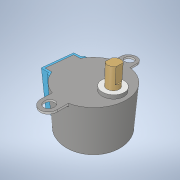
# Autodesk Inventor part: Stepper 28BYJ-48
Saved by Autodesk Inventor 2021.1 (Build 251245010, 245A)
## iProperties
Created: 2020-12-02
Part Number: Stepper 28BYJ-48
Material: Типовые
Document SubType Name: Modeling
Designer: Администратор
Density: 1 g/cm^3
Appearance: По умолчанию
Author: Администратор
Autodesk Inventor part; units mm, degrees
ref_plane "YZ Plane" through (0, 0, 0) normal (1, 0, 0) x (0, 1, 0)
ref_plane "XZ Plane" through (0, 0, 0) normal (0, 1, 0) x (-1, 0, 0)
ref_plane "XY Plane" through (0, 0, 0) normal (0, 0, 1) x (1, 0, 0)
sketch "Эскиз1" plane through (0, 0, 0) normal (0, 1, 0) x (-1, 0, 0)
  circle A0 centre (0, 0) radius 14
  dimension "d0" = 28
  constraints: 1 centre point, 1 coincident
  measures "d0" diameter of A0
extrude "Выдавливание1" add sketch "Эскиз1" along normal blind 19
sketch "Эскиз2" plane through (0, 19, 0) normal (0, 1, 0) x (1, 0, 0)
  circle A0 centre (8, 0) radius 4.5
  point P0 (0, 0)
  dimension "d3" = 9
  dimension "d4" = 8
  constraints: 1 centre point
  measures "d3" diameter of A0
  measures "d4" distance of point (0, 0) A0.centre
extrude "Выдавливание2" add sketch "Эскиз2" along normal blind 1.5
sketch "Эскиз3" plane through (8, 20.5, 0) normal (0, 1, 0) x (1, 0, 0)
  circle A0 centre (0, 0) radius 2.5
  point P0 (-8, 0)
  dimension "d7" = 5
  constraints: 1 centre point
  measures "d7" diameter of A0
extrude "Выдавливание3" add sketch "Эскиз3" along normal blind 8
sketch "Эскиз4" plane through (8, 28.5, 0) normal (0, 1, 0) x (1, 0, 0)
  circle A0 centre (0, 0) radius 2.5 projected
  line L0 (2, 1.5) -> (2, -1.5)
  line L1 (-2, -1.5) -> (-2, 1.5)
  point P0 (-8, 0)
  dimension "d12" = 3
  dimension "d13" = 3
  constraints: 4 end point, 4 point on circle, 1 parallel, 1 vertical
  measures "d12" distance of L0.start L0.end
  measures "d13" distance of L1.start L1.end
extrude "Выдавливание4" cut sketch "Эскиз4" against normal blind 6 contours A0 L0 | L1 A0
sketch "Эскиз5" plane through (0, 19, 0) normal (0, 1, 0) x (1, 0, 0)
  arc A0 (-3.5, -17.5) -> (3.5, -17.5) centre (0, -17.5) ccw
  arc A1 (3.5, 17.5) -> (-3.5, 17.5) centre (0, 17.5) ccw
  circle A2 centre (0, 0) radius 14 projected
  line L0 (-3.5, -17.5) -> (-3.5, -13.5554)
  line L1 (3.5, 17.5) -> (3.5, 13.5554)
  line L2 (-3.5, 17.5) -> (-3.5, 13.5554)
  line L3 (3.5, -17.5) -> (3.5, -13.5554)
  line L4 (0, 29.4009) -> (0, -29.4054) construction
  circle A3 centre (8, 0) radius 4.5 projected
  dimension "d16" = 7
  dimension "d17" = 17.5
  dimension "d18" = 7
  dimension "d19" = 17.5
  dimension "d41" = 8
  constraints: 10 point on circle, 8 end point, 4 point on line, 4 tangent, 3 vertical, 2 centre point, 1 parallel
  measures "d16" diameter of A0
  measures "d17" distance of point (0, 0) A0.centre
  measures "d18" diameter of A1
  measures "d19" distance of point (0, 0) A1.centre
  measures "d41" distance from line of A3.centre L4
extrude "Выдавливание5" add sketch "Эскиз5" against normal blind 0.8 contours L0 A2 L3 A0 | L2 A1 L1 A2
sketch "Эскиз6" plane through (0, 19, 0) normal (0, 1, 0) x (1, 0, 0)
  circle A0 centre (0, 17.5) radius 2.1
  circle A1 centre (0, -17.5) radius 2.1
  point P0 (0, 0)
  dimension "d22" = 4.2
  dimension "d23" = 4.2
  dimension "d24" = 17.5
  dimension "d25" = 17.5
  constraints: 2 centre point
  measures "d22" diameter of A0
  measures "d23" diameter of A1
  measures "d24" distance of point (0, 0) A0.centre
  measures "d25" distance of point (0, 0) A1.centre
extrude "Выдавливание6" cut sketch "Эскиз6" against normal blind 0.8
fillet "Сопряжение1" radius 0.5 1 edges at (14, 0, 0)
fillet "Сопряжение2" radius 0.5 1 edges at (0, 18.2, -14)
fillet "Сопряжение3" radius 0.5 1 edges at (0, 18.2, 14)
sketch "Эскиз7" plane through (0, 19, 0) normal (0, 1, 0) x (1, 0, 0)
  line L0 (-17, -7.3) -> (-17, 7.3)
  line L1 (0, 0) -> (-17, 0) construction
  line L2 (-13.1038, 7.3) -> (-17, 7.3)
  line L3 (-13.1038, -7.3) -> (-17, -7.3)
  arc A0 (-3.5, 13.5554) -> (-3.5, -13.5554) centre (0, 0) ccw projected
  line L4 (-12.5024, -6.3) -> (-16, -6.3)
  line L5 (-16, -6.3) -> (-16, 6.3)
  line L6 (-16, 6.3) -> (-12.5024, 6.3)
  line L7 (-11.2743, 8.3) -> (-12.4944, 8.3)
  line L8 (-12.4944, -8.3) -> (-11.2743, -8.3)
  arc A1 (-12.4944, 8.3) -> (-13.1038, 7.3) centre (0, 0) ccw
  arc A2 (-13.1038, -7.3) -> (-12.4944, -8.3) centre (0, 0) ccw
  point P0 (0, 7.4186)
  point P1 (0, -7.4186)
  point P2 (-11.9461, 7.3)
  point P3 (-11.9461, -7.3)
  dimension "d31" = 17
  dimension "d32" = 14.6
  dimension "d33" = 1
  dimension "d35" = 1
  constraints: 18 end point, 10 point on circle, 3 perpendicular, 2 centre point, 2 coincident, 2 symmetric about line, 1 midpoint, 1 vertical
  measures "d31" distance from line of L0 L1.start
  measures "d32" distance between parallel lines of L3 L2
  measures "d33" distance between parallel lines of L3 L4
  measures "d35" distance between parallel lines of L2 L7
extrude "Выдавливание7" add sketch "Эскиз7" against normal blind 17 separate body contours L0 L2 A1 L7 A0 L6 L5 L4 L8 A2 L3
sketch "Эскиз9" plane through (0, 19, 0) normal (0, 1, 0) x (1, 0, 0)
  arc A0 (-3.5, 13.5554) -> (-3.5, -13.5554) centre (0, 0) ccw projected
  line L0 (-3.5, 13.5554) -> (-3.5, 17.5) projected
  arc A1 (3.5, 17.5) -> (-3.5, 17.5) centre (0, 17.5) ccw projected
  line L1 (3.5, 17.5) -> (3.5, 13.5554) projected
  arc A2 (3.5, -13.5554) -> (3.5, 13.5554) centre (0, 0) ccw projected
  line L2 (3.5, -13.5554) -> (3.5, -17.5) projected
  arc A3 (-3.5, -17.5) -> (3.5, -17.5) centre (0, -17.5) ccw projected
  line L3 (-3.5, -17.5) -> (-3.5, -13.5554) projected
  circle A4 centre (0, 17.5) radius 2.1 projected
  circle A5 centre (0, -17.5) radius 2.1 projected
  circle A6 centre (8, 0) radius 4.5 projected
  arc A7 (-13.1038, -7.3) -> (-12.4944, -8.3) centre (0, 0) ccw projected
  line L4 (-13.1038, -7.3) -> (-17, -7.3) projected
  line L5 (-17, -7.3) -> (-17, 7.3) projected
  line L6 (-17, 7.3) -> (-13.1038, 7.3) projected
  arc A8 (-12.4944, 8.3) -> (-13.1038, 7.3) centre (0, 0) ccw projected
  line L7 (-12.4944, 8.3) -> (-11.2743, 8.3) projected
  arc A9 (-11.2743, 8.3) -> (-12.5024, 6.3) centre (0, 0) ccw projected
  line L8 (-12.5024, 6.3) -> (-16, 6.3) projected
  line L9 (-16, 6.3) -> (-16, -6.3) projected
  line L10 (-16, -6.3) -> (-12.5024, -6.3) projected
  arc A10 (-12.5024, -6.3) -> (-11.2743, -8.3) centre (0, 0) ccw projected
  line L11 (-11.2743, -8.3) -> (-12.4944, -8.3) projected
  arc A11 (-3.5, 13.5554) -> (-3.5, -13.5554) centre (0, 0) ccw projected
  line L12 (-3.5, 13.5554) -> (-3.5, 17.5) projected
  line L13 (-3.5, -17.5) -> (-3.5, -13.5554) projected
  circle A12 centre (0, 17.5) radius 2.1 projected
  circle A13 centre (0, -17.5) radius 2.1 projected
  circle A14 centre (8, 0) radius 4.5 projected
  arc A15 (-13.1038, -7.3) -> (-12.4944, -8.3) centre (0, 0) ccw projected
  line L14 (-13.1038, -7.3) -> (-17, -7.3) projected
  line L15 (-17, -7.3) -> (-17, 7.3) projected
  line L16 (-17, 7.3) -> (-13.1038, 7.3) projected
  arc A16 (-12.4944, 8.3) -> (-13.1038, 7.3) centre (0, 0) ccw projected
  line L17 (-12.4944, 8.3) -> (-11.2743, 8.3) projected
  arc A17 (-11.2743, 8.3) -> (-12.5024, 6.3) centre (0, 0) ccw projected
  line L18 (-12.5024, 6.3) -> (-16, 6.3) projected
  line L19 (-16, 6.3) -> (-16, -6.3) projected
  line L20 (-16, -6.3) -> (-12.5024, -6.3) projected
  arc A18 (-12.5024, -6.3) -> (-11.2743, -8.3) centre (0, 0) ccw projected
  line L21 (-11.2743, -8.3) -> (-12.4944, -8.3) projected
  arc A19 (-3.5, 13.5554) -> (-3.5, -13.5554) centre (0, 0) ccw projected
  line L22 (-3.5, 13.5554) -> (-3.5, 17.5) projected
  line L23 (-3.5, -17.5) -> (-3.5, -13.5554) projected
  circle A20 centre (0, 17.5) radius 2.1 projected
  circle A21 centre (0, -17.5) radius 2.1 projected
  circle A22 centre (8, 0) radius 4.5 projected
  arc A23 (-13.1038, -7.3) -> (-12.4944, -8.3) centre (0, 0) ccw projected
  line L24 (-13.1038, -7.3) -> (-17, -7.3) projected
  line L25 (-17, -7.3) -> (-17, 7.3) projected
  line L26 (-17, 7.3) -> (-13.1038, 7.3) projected
  arc A24 (-12.4944, 8.3) -> (-13.1038, 7.3) centre (0, 0) ccw projected
  line L27 (-12.4944, 8.3) -> (-11.2743, 8.3) projected
  arc A25 (-11.2743, 8.3) -> (-12.5024, 6.3) centre (0, 0) ccw projected
  line L28 (-12.5024, 6.3) -> (-16, 6.3) projected
  line L29 (-16, 6.3) -> (-16, -6.3) projected
  line L30 (-16, -6.3) -> (-12.5024, -6.3) projected
  arc A26 (-12.5024, -6.3) -> (-11.2743, -8.3) centre (0, 0) ccw projected
  line L31 (-11.2743, -8.3) -> (-12.4944, -8.3) projected
  arc A27 (-3.5, 13.5554) -> (-3.5, -13.5554) centre (0, 0) ccw projected
  line L32 (-3.5, 13.5554) -> (-3.5, 17.5) projected
  line L33 (-3.5, -17.5) -> (-3.5, -13.5554) projected
  circle A28 centre (0, 17.5) radius 2.1 projected
  circle A29 centre (0, -17.5) radius 2.1 projected
  circle A30 centre (8, 0) radius 4.5 projected
  arc A31 (-13.1038, -7.3) -> (-12.4944, -8.3) centre (0, 0) ccw projected
  line L34 (-13.1038, -7.3) -> (-17, -7.3) projected
  line L35 (-17, -7.3) -> (-17, 7.3) projected
  line L36 (-17, 7.3) -> (-13.1038, 7.3) projected
  arc A32 (-12.4944, 8.3) -> (-13.1038, 7.3) centre (0, 0) ccw projected
  line L37 (-12.4944, 8.3) -> (-11.2743, 8.3) projected
  arc A33 (-11.2743, 8.3) -> (-12.5024, 6.3) centre (0, 0) ccw projected
  line L38 (-12.5024, 6.3) -> (-16, 6.3) projected
  line L39 (-16, 6.3) -> (-16, -6.3) projected
  line L40 (-16, -6.3) -> (-12.5024, -6.3) projected
  arc A34 (-12.5024, -6.3) -> (-11.2743, -8.3) centre (0, 0) ccw projected
  line L41 (-11.2743, -8.3) -> (-12.4944, -8.3) projected
  arc A35 (-3.5, 13.5554) -> (-3.5, -13.5554) centre (0, 0) ccw projected
  line L42 (-16, 6.3) -> (-12.5024, 6.3) projected
  line L43 (-16, -6.3) -> (-16, 6.3) projected
  circle A36 centre (0, 17.5) radius 2.1 projected
  circle A37 centre (0, -17.5) radius 2.1 projected
  circle A38 centre (8, 0) radius 4.5 projected
  arc A39 (-3.5, 13.5554) -> (-3.5, -13.5554) centre (0, 0) ccw projected
  line L44 (-3.5, -13.5554) -> (-3.5, -17.5) projected
  arc A40 (-3.5, -17.5) -> (3.5, -17.5) centre (0, -17.5) ccw projected
  line L45 (3.5, -17.5) -> (3.5, -13.5554) projected
  arc A41 (3.5, -13.5554) -> (3.5, 13.5554) centre (0, 0) ccw projected
  line L46 (3.5, 13.5554) -> (3.5, 17.5) projected
  arc A42 (3.5, 17.5) -> (-3.5, 17.5) centre (0, 17.5) ccw projected
  line L47 (-3.5, 17.5) -> (-3.5, 13.5554) projected
  arc A43 (-3.5, 13.5554) -> (-3.5, -13.5554) centre (0, 0) ccw projected
  line L48 (-3.5, 13.5554) -> (-3.5, 17.5) projected
  line L49 (-3.5, -17.5) -> (-3.5, -13.5554) projected
  circle A44 centre (0, 17.5) radius 2.1 projected
  circle A45 centre (0, -17.5) radius 2.1 projected
  circle A46 centre (8, 0) radius 4.5 projected
  arc A47 (-13.1038, -7.3) -> (-12.4944, -8.3) centre (0, 0) ccw projected
  line L50 (-13.1038, -7.3) -> (-17, -7.3) projected
  line L51 (-17, -7.3) -> (-17, 7.3) projected
  line L52 (-17, 7.3) -> (-13.1038, 7.3) projected
  arc A48 (-12.4944, 8.3) -> (-13.1038, 7.3) centre (0, 0) ccw projected
  line L53 (-12.4944, 8.3) -> (-11.2743, 8.3) projected
  arc A49 (-11.2743, 8.3) -> (-12.5024, 6.3) centre (0, 0) ccw projected
  line L54 (-12.5024, 6.3) -> (-16, 6.3) projected
  line L55 (-16, 6.3) -> (-16, -6.3) projected
  line L56 (-16, -6.3) -> (-12.5024, -6.3) projected
  arc A50 (-12.5024, -6.3) -> (-11.2743, -8.3) centre (0, 0) ccw projected
  line L57 (-11.2743, -8.3) -> (-12.4944, -8.3) projected
  arc A51 (3.5, 17.5) -> (-3.5, 17.5) centre (0, 17.5) ccw projected
  line L58 (3.5, 17.5) -> (3.5, 13.5554) projected
  arc A52 (3.5, -13.5554) -> (3.5, 13.5554) centre (0, 0) ccw projected
  line L59 (3.5, -13.5554) -> (3.5, -17.5) projected
  arc A53 (-3.5, -17.5) -> (3.5, -17.5) centre (0, -17.5) ccw projected
  arc A54 (3.5, 17.5) -> (-3.5, 17.5) centre (0, 17.5) ccw projected
  line L60 (3.5, 17.5) -> (3.5, 13.5554) projected
  arc A55 (3.5, -13.5554) -> (3.5, 13.5554) centre (0, 0) ccw projected
  line L61 (3.5, -13.5554) -> (3.5, -17.5) projected
  arc A56 (-3.5, -17.5) -> (3.5, -17.5) centre (0, -17.5) ccw projected
  arc A57 (3.5, 17.5) -> (-3.5, 17.5) centre (0, 17.5) ccw projected
  line L62 (3.5, 17.5) -> (3.5, 13.5554) projected
  arc A58 (3.5, -13.5554) -> (3.5, 13.5554) centre (0, 0) ccw projected
  line L63 (3.5, -13.5554) -> (3.5, -17.5) projected
  arc A59 (-3.5, -17.5) -> (3.5, -17.5) centre (0, -17.5) ccw projected
  arc A60 (3.5, 17.5) -> (-3.5, 17.5) centre (0, 17.5) ccw projected
  line L64 (3.5, 17.5) -> (3.5, 13.5554) projected
  arc A61 (3.5, -13.5554) -> (3.5, 13.5554) centre (0, 0) ccw projected
  line L65 (3.5, -13.5554) -> (3.5, -17.5) projected
  arc A62 (-3.5, -17.5) -> (3.5, -17.5) centre (0, -17.5) ccw projected
extrude "Выдавливание8" add sketch "Эскиз9" against normal blind 17 contours A0 L10 L9 L8 bodies 1
fillet "Сопряжение4" radius 0.3 1 edges at (-17, 10.5, 7.3)
